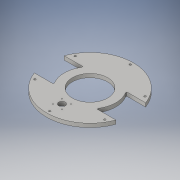
# Autodesk Inventor part: Turntable Mount
Saved by Autodesk Inventor 2016 (Build 200138000, 138)
## iProperties
Created: 2016-04-25
Part Number: Turntable Mount
Material: Generic
Document SubType Name: Modeling
Designer: rubenjm
Density: 1 g/cm^3
Appearance: Default
Author: rubenjm
Autodesk Inventor part; units mm, degrees
ref_plane "YZ Plane" through (0, 0, 0) normal (1, 0, 0) x (0, 1, 0)
ref_plane "XZ Plane" through (0, 0, 0) normal (0, 1, 0) x (-1, 0, 0)
ref_plane "XY Plane" through (0, 0, 0) normal (0, 0, 1) x (1, 0, 0)
sketch "Sketch1" plane through (0, 0, 0) normal (0, 1, 0) x (-1, 0, 0)
  circle A0 centre (0, 0) radius 60.325
  circle A1 centre (0, 0) radius 148.0058
  line L0 (0, 0) -> (-122.3635, 70.6466) construction
  line L1 (0, 0) -> (141.2932, 0) construction
  line L2 (-122.3635, 70.6466) -> (0, 0) construction
  line L3 (0, 0) -> (-128.1768, -74.0029) construction
  circle A2 centre (0, 0) radius 148.0058 construction
  line L4 (0, 0) -> (148.0058, 0) construction
  circle A3 centre (0, 0) radius 137.541 construction
  circle A4 centre (-119.114, -68.7705) radius 3.175
  circle A5 centre (0, -137.541) radius 3.175
  circle A6 centre (119.114, -68.7705) radius 3.175
  circle A7 centre (119.114, 68.7705) radius 3.175
  circle A8 centre (0, 137.541) radius 3.175
  circle A9 centre (-119.114, 68.7705) radius 3.175
  dimension "d22" = 275.082
  dimension "d16" = 120.65
  dimension "d17" = 296.0116
  dimension "d20" = 150
  dimension "d21" = 150
  dimension "d23" = 6.35
  dimension "d24" = 360
  constraints: 10 end point, 8 centre point, 3 coincident, 2 equal length, 2 horizontal, 1 collinear, 1 point on line, 19 other
  measures "d16" diameter of A0
  measures "d17" diameter of A1
  measures "d20" angle of L1 L0
  measures "d21" angle of L3 L4
  measures "d23" diameter of A4
extrude "Extrusion1" add sketch "Sketch1" along normal blind 12.7
sketch "Sketch2" plane through (0, 12.7, 0) normal (0, 1, 0) x (1, 0, 0)
  circle A0 centre (0, 0) radius 119.634 construction
  line L0 (-0.0021, -119.634) -> (-0.0021, -118.8974) construction
  line L1 (-0.0021, -119.634) -> (0.7345, -119.634) construction
  line L2 (-0.0021, -118.8974) -> (-0.0021, -113.6396) construction
  line L3 (-0.0021, -118.8974) -> (5.2557, -118.8974) construction
  line L4 (-21.15, -80.1691) -> (-21.15, -111.1691) construction
  line L5 (15.5, -116.8191) -> (-15.5, -116.8191) construction
  line L6 (21.15, -111.1691) -> (21.15, -80.1691) construction
  line L7 (-15.5, -74.5191) -> (15.5, -74.5191) construction
  line L8 (15.5, -74.5191) -> (21.15, -80.1691) construction
  line L9 (21.15, -111.1691) -> (15.5, -116.8191) construction
  line L10 (-15.5, -116.8191) -> (-21.15, -111.1691) construction
  line L11 (-21.15, -80.1691) -> (-15.5, -74.5191) construction
  line L12 (-15.5, -111.1691) -> (15.5, -111.1691) construction
  line L13 (15.5, -111.1691) -> (15.5, -80.1691) construction
  line L14 (15.5, -80.1691) -> (-15.5, -80.1691) construction
  line L15 (-15.5, -80.1691) -> (-15.5, -111.1691) construction
  line L16 (-15.5, -111.1691) -> (15.5, -80.1691) construction
  line L17 (15.5, -111.1691) -> (-15.5, -80.1691) construction
  circle A1 centre (15.5, -80.1691) radius 1.5
  circle A2 centre (15.5, -111.1691) radius 1.5
  circle A3 centre (-15.5, -111.1691) radius 1.5
  circle A4 centre (-15.5, -80.1691) radius 1.5
  circle A5 centre (0, -95.6691) radius 11.049
  dimension "d27" = 239.268
  dimension "d28" = 0.7366
  dimension "d29" = 90
  dimension "d30" = 5.2578
  dimension "d31" = 90
  dimension "d32" = 3
  dimension "d33" = 3
  dimension "d34" = 3
  dimension "d35" = 22.098
  constraints: 36 end point, 5 centre point, 4 perpendicular, 3 coincident, 3 horizontal, 2 midpoint, 2 parallel, 2 vertical, 3 other
  measures "d28" distance of L0.start L0.end
  measures "d29" angle of L1 L0
  measures "d30" distance of L0.end L2.end
  measures "d31" angle of L3 L2
  measures "d32" diameter of A1
  measures "d33" diameter of A3
  measures "d34" diameter of A4
  measures "d35" diameter of A5
extrude "Extrusion2" cut sketch "Sketch2" against normal through all
sketch "Sketch3" plane through (0, 12.7, 0) normal (0, 1, 0) x (1, 0, 0)
  line L0 (-148.0058, 50.8) -> (-148.0058, -50.8)
  line L1 (148.0058, -50.8) -> (148.0058, 50.8)
  line L2 (148.0058, 50.8) -> (-148.0058, -50.8) construction
  line L3 (-148.0058, 50.8) -> (148.0058, -50.8) construction
  line L4 (75.193, -50.8) -> (-75.193, 50.8) construction
  line L5 (-75.193, -50.8) -> (75.193, 50.8) construction
  line L6 (-148.0058, -50.8) -> (-75.193, -50.8)
  line L7 (75.193, -50.8) -> (148.0058, -50.8)
  line L8 (148.0058, 50.8) -> (75.193, 50.8)
  line L9 (-75.193, 50.8) -> (-148.0058, 50.8)
  line L10 (-75.193, -50.8) -> (-75.193, -45.7676)
  line L11 (-75.193, 45.7676) -> (-75.193, 50.8)
  line L12 (75.193, 50.8) -> (75.193, 45.7676)
  line L13 (75.193, -45.7676) -> (75.193, -50.8)
  arc A0 (75.193, -45.7676) -> (75.193, 45.7676) centre (0, 0) ccw
  arc A1 (-75.193, 45.7676) -> (-75.193, -45.7676) centre (0, 0) ccw
  dimension "d38" = 296.0116
  dimension "d39" = 101.6
  constraints: 28 end point, 9 parallel, 4 midpoint, 4 point on circle, 2 centre point, 2 horizontal, 2 perpendicular, 1 coincident
  measures "d38" distance of L1.start L0.end
  measures "d39" distance of L0.end L0.start
extrude "Extrusion4" cut sketch "Sketch3" against normal through all
body "Solid1"
